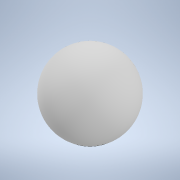
# Autodesk Inventor part: Деталь6
Saved by Autodesk Inventor 2021.1 (Build 251245010, 245A)
## iProperties
Created: 2023-09-28
Part Number: Деталь6
Material: Типовые
Document SubType Name: Modeling
Designer: Lenovo
Density: 1 g/cm^3
Appearance: По умолчанию
Author: Lenovo
Autodesk Inventor part; units mm, degrees
ref_plane "YZ Plane" through (0, 0, 0) normal (1, 0, 0) x (0, 1, 0)
ref_plane "XZ Plane" through (0, 0, 0) normal (0, 1, 0) x (-1, 0, 0)
ref_plane "XY Plane" through (0, 0, 0) normal (0, 0, 1) x (1, 0, 0)
sketch "Эскиз2" plane through (0, 0, 0) normal (0, 0, 1) x (1, 0, 0)
  arc A0 (358.9749, 18.5) -> (354, 35) centre (354, 26) ccw
  line L0 (354, 35) -> (354, 22.2)
  line L1 (354, 22.2) -> (356, 22.2)
  line L2 (356, 22.2) -> (356, 18.5)
  line L3 (356, 18.5) -> (358.9749, 18.5)
  point P0 (0, 0)
  dimension "d17" = 16.5
  constraints: 8 end point, 2 perpendicular, 2 point on circle, 1 centre point, 1 horizontal, 1 vertical
  measures "d17" vertical distance of L3.end L0.start
revolve "Вращение1" add sketch "Эскиз2" angle 360 about axis through (354, 35, 0) along (0, -1, 0)
